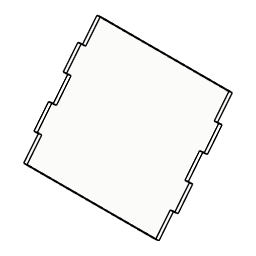
smartie_slide (Autodesk Fusion 360 archive; units mm, degrees)
design "Slide Panel"
part number: 2025-05-20-12-54-31-195
Autodesk Fusion 360 part; units mm, degrees
sketch "Slide" plane through (0, 0, 0) normal (1, 0, 0) x (0, 1, 0)
  line L0 (0, 0) -> (49.9812, 62.4765)
  line L1 (49.9812, 62.4765) -> (52.3238, 60.6024)
  line L2 (0, 0) -> (2.3426, -1.8741)
  line L3 (2.3426, -1.8741) -> (52.3238, 60.6024)
  dimension "d2" = 80.009
  dimension "d3" = 3
  dimension "d4" = 3
  constraint coincident L0.start L2.start
  constraint perpendicular L0 L1
  constraint perpendicular L0 L2
  measures "d2" distance of L0.start L0.end
  measures "d3" distance of L0.end L1.end
  measures "d4" distance of L0.start L2.end
extrude "Extrude1" add sketch "Slide" against normal blind 96
sketch "Top" plane through (0, 0, 0) normal (0, -0.780869, 0.624695) x (1, 0, 0)
  line L0 (0, 0) -> (0, 80.009)
  line L1 (0, 80.009) -> (-96, 80.009)
  line L2 (-96, 80.009) -> (-96, 0)
  line L3 (-96, 0) -> (0, 0)
  line L4 (0, 80.009) -> (-3, 80.009)
  line L5 (-3, 80.009) -> (-3, 64.009)
  line L6 (-3, 64.009) -> (0, 64.009)
  line L7 (0, 64.009) -> (0, 80.009)
  line L8 (0, 48.009) -> (-3, 48.009)
  line L9 (-3, 48.009) -> (-3, 32.009)
  line L10 (-3, 32.009) -> (0, 32.009)
  line L11 (0, 32.009) -> (0, 48.009)
  line L12 (0, 16) -> (-3, 16)
  line L13 (-3, 16) -> (-3, 0)
  line L14 (-3, 0) -> (0, 0)
  line L15 (0, 0) -> (0, 16)
  line L16 (-96, 80.009) -> (-93, 80.009)
  line L17 (-93, 80.009) -> (-93, 64.009)
  line L18 (-93, 64.009) -> (-96, 64.009)
  line L19 (-96, 64.009) -> (-96, 80.009)
  line L20 (-96, 48.009) -> (-93, 48.009)
  line L21 (-93, 48.009) -> (-93, 32.009)
  line L22 (-93, 32.009) -> (-96, 32.009)
  line L23 (-96, 32.009) -> (-96, 48.009)
  line L24 (-96, 16) -> (-93, 16)
  line L25 (-93, 16) -> (-93, 0)
  line L26 (-93, 0) -> (-96, 0)
  line L27 (-96, 0) -> (-96, 16)
  dimension "d7" = 3
  dimension "d8" = 16
  dimension "d9" = 16
  dimension "d10" = 16
  dimension "d11" = 16
  dimension "d12" = 16.009
  dimension "d13" = 3
  dimension "d14" = 16
  dimension "d15" = 16
  dimension "d16" = 16
  dimension "d17" = 16
  dimension "d18" = 16.009
  constraint horizontal L4
  constraint vertical L5
  constraint horizontal L6
  constraint vertical L7
  constraint coincident L0.end L1.start
  constraint horizontal L8
  constraint vertical L9
  constraint horizontal L10
  constraint vertical L11
  constraint coincident L0 L8.start
  constraint horizontal L12
  constraint vertical L13
  constraint horizontal L14
  constraint vertical L15
  constraint coincident L3 L13.end
  constraint coincident L0 L12.start
  constraint collinear L5 L9
  constraint collinear L9 L13
  constraint horizontal L16
  constraint vertical L17
  constraint horizontal L18
  constraint vertical L19
  constraint coincident L1.end L2.start
  constraint horizontal L20
  constraint vertical L21
  constraint horizontal L22
  constraint vertical L23
  constraint coincident L2 L20.start
  constraint horizontal L24
  constraint vertical L25
  constraint horizontal L26
  constraint vertical L27
  constraint coincident L3 L25.end
  constraint coincident L2 L24.start
  constraint collinear L17 L21
  constraint collinear L21 L25
  measures "d7" distance of L5 L7
  measures "d8" distance of L0.end L6.end
  measures "d9" distance of L8.start L10.end
  measures "d10" distance of L6 L8
  measures "d11" distance of L12.start L0.start
  measures "d12" distance of L10 L12
  measures "d13" distance of L1.end L16.end
  measures "d14" distance of L1.end L18.end
  measures "d15" distance of L20.start L22.end
  measures "d16" distance of L24.start L2.end
  measures "d17" distance of L18 L20
  measures "d18" distance of L22 L24
extrude "Extrude2" cut sketch "Top" against normal blind 3 contours L0 L3 L12 L13 L14 L15 | L0 L8 L9 L10 L11 | L2 L3 L24 L25 L26 L27 | L0 L1 L4 L5 L6 L7 | L2 L20 L21 L22 L23 | L1 L2 L16 L17 L18 L19
equation "acrylic_thickness = 3 mm" comment "Thickness of the clear acrylic panels."
equation "d3 = acrylic_thickness"
equation "d4 = acrylic_thickness"
equation "d7 = acrylic_thickness"
equation "d13 = acrylic_thickness"
equation "d19 = -acrylic_thickness"
named bodies: "Slide Panel"
